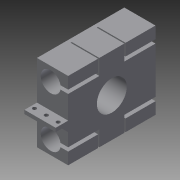
# Autodesk Inventor part: XCarriage
Saved by Autodesk Inventor 2015 (Build 190159000, 159)
## iProperties
Created: 2014-08-17
Part Number: XCarriage
Material: Generic
Document SubType Name: Modeling
Designer: Jack
Density: 1 g/cm^3
Appearance: Default
Author: Jack
Autodesk Inventor part; units mm, degrees
ref_plane "YZ Plane" through (0, 0, 0) normal (1, 0, 0) x (0, 1, 0)
ref_plane "XZ Plane" through (0, 0, 0) normal (0, 1, 0) x (-1, 0, 0)
ref_plane "XY Plane" through (0, 0, 0) normal (0, 0, 1) x (1, 0, 0)
sketch "Sketch8" plane through (0, 0, 0) normal (0, 1, 0) x (-1, 0, 0)
  arc A0 (-7.8581, -1.5) -> (-7.8581, 1.5) centre (0, 0) ccw
  arc A1 (-7.8581, -41.5) -> (-7.8581, -38.5) centre (0, -40) ccw
  line L0 (11, 11) -> (-14, 11)
  line L1 (11, 11) -> (11, -51)
  line L2 (11, -51) -> (-14, -51)
  line L3 (-14, 11) -> (-14, 1.5)
  line L4 (-14, 1.5) -> (-7.8581, 1.5)
  line L5 (-7.8581, -1.5) -> (-14, -1.5)
  line L6 (-14, -1.5) -> (-14, -38.5)
  line L7 (-14, -38.5) -> (-7.8581, -38.5)
  line L8 (-7.8581, -41.5) -> (-14, -41.5)
  line L9 (-14, -41.5) -> (-14, -51)
  dimension "d27" = 16
  dimension "d28" = 16
  dimension "d29" = 40
  dimension "d30" = 11
  dimension "d31" = 11
  dimension "d32" = 11
  dimension "d33" = 1.5
  dimension "d34" = 1.5
  dimension "d35" = 1.5
  dimension "d36" = 1.5
  dimension "d37" = 14
  constraints: 20 end point, 5 perpendicular, 4 point on circle, 3 horizontal, 3 vertical alignment, 2 centre point, 2 vertical, 1 coincident
  measures "d27" diameter of A0
  measures "d28" diameter of A1
  measures "d29" distance of point (0, 0) A1.centre
  measures "d30" distance from line of point (0, 0) L1
  measures "d31" distance from line of point (0, 0) L0
  measures "d32" distance from line of L2 A1.centre
  measures "d33" distance from line of A1.centre L8
  measures "d34" distance from line of A1.centre L7
  measures "d35" distance from line of point (0, 0) L5
  measures "d36" distance from line of A0.centre L4
  measures "d37" distance from line of point (0, 0) L3
extrude "Extrusion5" add sketch "Sketch8" along normal blind 70
ref_plane "Work Plane3" through (0, 45, 0) normal (0, 1, 0) x (1, 0, 0)
ref_plane "Work Plane4" through (0, 25, 0) normal (0, -1, 0) x (1, 0, 0)
sketch "Sketch9" plane through (0, 45, 0) normal (0, 1, 0) x (1, 0, 0)
  circle A0 centre (0, 0) radius 8
  arc A1 (7.8581, 41.5) -> (7.8581, 38.5) centre (0, 40) ccw projected
  circle A2 centre (0, 40) radius 8
  dimension "d42" = 16
  constraints: 2 centre point, 2 coincident, 1 concentric
  measures "d42" diameter of A0
extrude "Extrusion6" add sketch "Sketch9" against normal blind 20
sketch "Sketch14" plane through (14, 0, -51) normal (0, 0, -1) x (-1, 0, 0)
  line L0 (0, 0) -> (25, 0) projected
  line L1 (0, 70) -> (25, 70) projected
  line L2 (0, 0) -> (0, 70) projected
  line L3 (0, 46) -> (22, 46)
  line L4 (22, 46) -> (22, 45)
  line L5 (22, 45) -> (0, 45)
  line L6 (0, 45) -> (0, 46)
  line L7 (0, 0) -> (0, 70) projected
  line L8 (0, 25) -> (22, 25)
  line L9 (22, 25) -> (22, 24)
  line L10 (22, 24) -> (0, 24)
  line L11 (0, 24) -> (0, 25)
  point P0 (14, 0)
  dimension "d61" = 22
  dimension "d62" = 1
  dimension "d63" = 24
  dimension "d64" = 22
  dimension "d65" = 1
  dimension "d66" = 24
  constraints: 16 end point, 6 perpendicular, 4 point on line, 2 horizontal, 1 collinear
  measures "d61" distance of L3.start L3.end
  measures "d62" distance of L3.end L4.end
  measures "d63" distance between parallel lines of L1 L3
  measures "d64" distance of L8.start L8.end
  measures "d65" distance of L8.end L9.end
  measures "d66" distance between parallel lines of L0 L10
extrude "Extrusion9" cut sketch "Sketch14" against normal blind 11
sketch "Sketch15" plane through (7.8581, 25, -41.5) normal (0, 0, 1) x (1, 0, 0)
  line L0 (0, 0) -> (6.1419, 0) projected
  line L1 (6.1419, 0) -> (6.1419, 20) projected
  line L2 (6.1419, 20) -> (0, 20) projected
  line L3 (0, 0) -> (0, 20) projected
  point P0 (-7.8581, -25)
extrude "Extrusion10" add sketch "Sketch15" along normal up to surface (3 mm away)
sketch "Sketch16" plane through (-11, 0, 11) normal (0, 0, 1) x (1, 0, 0)
  line L0 (0, 0) -> (25, 0) projected
  line L1 (0, 70) -> (25, 70) projected
  line L2 (25, 0) -> (25, 25) projected
  line L3 (25, 24) -> (3, 24)
  line L4 (3, 24) -> (3, 25)
  line L5 (3, 25) -> (25, 25)
  line L6 (25, 25) -> (25, 24)
  line L7 (25, 46) -> (25, 70) projected
  line L8 (25, 46) -> (3, 46)
  line L9 (3, 46) -> (3, 45)
  line L10 (3, 45) -> (25, 45)
  line L11 (25, 45) -> (25, 46)
  point P0 (11, 0)
  dimension "d71" = 22
  dimension "d72" = 1
  dimension "d73" = 22
  dimension "d74" = 1
  dimension "d75" = 24
  dimension "d76" = 24
  constraints: 16 end point, 4 parallel, 2 horizontal, 2 perpendicular, 2 point on line
  measures "d71" distance of L4.end L5.end
  measures "d72" distance of L3.end L4.end
  measures "d73" distance of L10.end L9.end
  measures "d74" distance of L9.end L8.end
  measures "d75" distance between parallel lines of L0 L3
  measures "d76" distance between parallel lines of L1 L8
extrude "Extrusion11" cut sketch "Sketch16" against normal blind 11
sketch "Sketch17" plane through (14, 25, 1.5) normal (0, 0, -1) x (-1, 0, 0)
  line L0 (0, 0) -> (6.1419, 0) projected
  line L1 (6.1419, 0) -> (6.1419, 20) projected
  line L2 (6.1419, 20) -> (0, 20) projected
  line L3 (0, 0) -> (0, 20) projected
  point P0 (14, -25)
extrude "Extrusion12" add sketch "Sketch17" along normal up to surface (3 mm away)
sketch "Sketch18" plane through (-11, 0, -51) normal (-1, 0, 0) x (0, 0, 1)
  line L0 (0, 70) -> (62, 70) projected
  line L1 (0, 0) -> (0, 70) projected
  circle A0 centre (31, 35) radius 12
  point P0 (51, 0)
  dimension "d81" = 24
  dimension "d82" = 35
  dimension "d83" = 31
  constraints: 1 centre point
  measures "d81" diameter of A0
  measures "d82" distance from line of L0 A0.centre
  measures "d83" distance from line of L1 A0.centre
extrude "Extrusion13" cut sketch "Sketch18" against normal up to surface (25 mm away)
sketch "Sketch19" plane through (0, 0, 0) normal (0, -1, 0) x (1, 0, 0)
  line L0 (-11, -51) -> (-11, 11) projected
  line L1 (14, -1.5) -> (14, -38.5) projected
  line L2 (14, -23) -> (-11, -23)
  line L3 (14, -20) -> (-11, -20)
  dimension "d86" = 3
  constraints: 4 end point, 2 midpoint, 2 point on line, 1 perpendicular
  measures "d86" distance between parallel lines of L2 L3
extrude "Extrusion14" add sketch "Sketch19" along normal blind 10
chamfer "Chamfer1" distance 5 angle 45 1 edges at (1.5, 0, -23)
sketch "Sketch20" plane through (-11, 0, -20) normal (0, 0, 1) x (1, 0, 0)
  line L0 (0, 0) -> (0, -10) projected
  line L1 (25, -10) -> (0, -10) projected
  line L2 (25, 0) -> (25, -10) projected
  circle A0 centre (3, -5) radius 1.5
  circle A1 centre (12.5, -5) radius 1.5
  circle A2 centre (22, -5) radius 1.5
  point P0 (11, 0)
  dimension "d92" = 3
  dimension "d93" = 3
  dimension "d94" = 3
  dimension "d95" = 3
  dimension "d96" = 3
  dimension "d97" = 5
  dimension "d98" = 9.5
  constraints: 3 centre point, 2 horizontal alignment
  measures "d92" diameter of A0
  measures "d93" diameter of A1
  measures "d94" diameter of A2
  measures "d95" distance from line of L2 A2.centre
  measures "d96" distance from line of L0 A0.centre
  measures "d97" distance from line of L1 A0.centre
  measures "d98" distance of A0.centre A1.centre
extrude "Extrusion15" cut sketch "Sketch20" against normal blind 4.75
body "Solid2"
